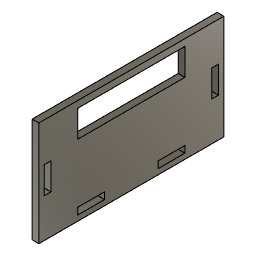
Drawer Front (Autodesk Fusion 360 design; units mm, degrees)
Autodesk Fusion 360 part; units mm, degrees
note: some values were not read from the file. Set by a fixed rule: which sketch regions a step uses.
sketch "Sketch1" plane through (0, 0, 0) normal (1, 0, 0) x (0, 1, 0)
  line L0 (25.4, 0) -> (25.4, -3.175)
  line L1 (12.7, 0) -> (12.7, -3.175)
  line L2 (76.2, 25.4) -> (76.2, 12.7)
  line L3 (0, 0) -> (0, 25.4)
  line L4 (0, 12.7) -> (-3.175, 12.7)
  line L5 (76.2, 12.7) -> (79.375, 12.7)
  line L6 (-3.175, 25.4) -> (0, 25.4)
  line L7 (63.5, -3.175) -> (63.5, 0)
  line L8 (50.8, 0) -> (50.8, -3.175)
  line L9 (79.375, 12.7) -> (79.375, 25.4)
  line L10 (0, -3.175) -> (0, 0)
  line L11 (0, 0) -> (0, 12.7)
  line L12 (25.4, -3.175) -> (38.1, -3.175)
  line L13 (-3.175, 12.7) -> (-3.175, 25.4)
  line L14 (79.375, 25.4) -> (76.2, 25.4)
  line L15 (0, 0) -> (-7.62, 0)
  line L16 (0, 0) -> (-5.715, 0)
  line L17 (-5.715, 0) -> (-5.715, 38.1)
  line L18 (-5.715, 38.1) -> (-5.715, 43.815)
  line L19 (-5.715, 43.815) -> (76.2, 43.815)
  line L20 (76.2, 43.815) -> (81.915, 43.815)
  line L21 (81.915, 43.815) -> (81.915, 0)
  line L22 (81.915, 0) -> (81.915, -5.715)
  line L23 (81.915, -5.715) -> (0, -5.715)
  line L24 (0, -5.715) -> (-5.715, -5.715)
  line L25 (-5.715, -5.715) -> (-5.715, 0)
  line L26 (-5.715, 43.815) -> (12.7, 43.815)
  line L27 (12.7, 43.815) -> (12.7, 40.64)
  line L28 (12.7, 40.64) -> (12.7, 27.94)
  line L29 (81.915, 43.815) -> (63.5, 43.815)
  line L30 (63.5, 43.815) -> (63.5, 27.94)
  line L31 (63.5, 27.94) -> (12.7, 27.94)
  line L32 (12.7, 40.64) -> (63.5, 40.64)
  line L33 (63.5, -3.175) -> (50.8, -3.175)
  line L34 (63.5, 0) -> (50.8, 0)
  line L35 (25.4, -3.175) -> (12.7, -3.175)
  line L36 (12.7, 0) -> (25.4, 0)
  dimension "d2" = 12.7
  dimension "d3" = 3.175
  dimension "d4" = 12.7
  dimension "d6" = 12.7
  dimension "d9" = 12.7
  dimension "d10" = 3.175
  dimension "d12" = 12.7
  dimension "d13" = 3.175
  dimension "d14" = 12.7
  dimension "d16" = 3.175
  dimension "d17" = 12.7
  dimension "d18" = 7.62
  dimension "d21" = 5.715
  dimension "d22" = 5.715
  dimension "d23" = 5.715
  dimension "d24" = 5.715
  dimension "d25" = 3.175
  dimension "d26" = 12.7
  dimension "d27" = 18.415
  constraint coincident L3.start L10.end
  constraint perpendicular L0 L12
  constraint perpendicular L3 L4
  constraint perpendicular L4 L13
  constraint perpendicular L3 L6
  constraint perpendicular L2 L5
  constraint perpendicular L5 L9
  constraint perpendicular L2 L14
  constraint perpendicular L3 L15
  constraint perpendicular L3 L16
  constraint perpendicular L15 L17
  constraint perpendicular L15 L18
  constraint perpendicular L18 L19
  constraint perpendicular L18 L20
  constraint perpendicular L20 L21
  constraint perpendicular L20 L22
  constraint perpendicular L22 L23
  constraint perpendicular L22 L24
  constraint perpendicular L15 L25
  constraint coincident L19 L26.end
  constraint perpendicular L18 L26
  constraint perpendicular L26 L27
  constraint parallel L27 L28
  constraint perpendicular L21 L29
  constraint perpendicular L19 L30
  constraint coincident L30 L32.end
  constraint perpendicular L30 L32
  constraint perpendicular L8 L33
  constraint perpendicular L8 L34
  constraint perpendicular L1 L35
  constraint perpendicular L0 L36
  measures "d2" distance of L1.start L3.start
  measures "d3" distance of L1.start L1.end
  measures "d4" distance of L1.start L0.start
  measures "d6" distance of L0.end L12.end
  measures "d9" distance of L7.end L8.start
  measures "d10" distance of L8.start L8.end
  measures "d12" distance of L3.start L4.start
  measures "d13" distance of L4.end L4.start
  measures "d14" distance of L6.start L4.end
  measures "d16" distance of L5.end L2.end
  measures "d17" distance of L5.end L9.end
  measures "d18" distance of L3.start L15.end
  measures "d21" distance of L3.start L16.end
  measures "d22" distance of L17.end L18.end
  measures "d23" distance of L19.end L20.end
  measures "d24" distance of L21.end L22.end
  measures "d25" distance of L26.end L27.end
  measures "d26" distance of L27.end L28.end
  measures "d27" distance of L20.end L29.end
extrude "Extrude1" add sketch "Sketch1" along normal blind 3.175 contours L17 L18 L19 L20 L21 L22 L23 L24 L25 L26 L27 L28 L29 L30 L31 | L19 L27 L30 L32
